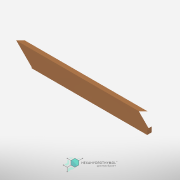
# Autodesk Inventor part: MPX-rib2
Saved by Autodesk Inventor 2016 (Build 200138000, 138)
## iProperties
Created: 2015-05-27
Part Number: MPX-rib2
Material: Wood (Cherry)
Document SubType Name: Modeling
Designer: as
Mass: 792.477 g
Surface Area: 1559.2 cm^2
Volume: 1257.9 cm^3
Density: 0.63 g/cm^3
Appearance: Cherry - Natural Low Gloss
Author: as
Autodesk Inventor part; units mm, degrees
ref_plane "YZ Plane" through (0, 0, 0) normal (1, 0, 0) x (0, 1, 0)
ref_plane "XZ Plane" through (0, 0, 0) normal (0, 1, 0) x (-1, 0, 0)
ref_plane "XY Plane" through (0, 0, 0) normal (0, 0, 1) x (1, 0, 0)
sketch "Sketch1" plane through (0, 0, 0) normal (0, 0, 1) x (1, 0, 0)
  line L0 (0, 0) -> (780, 0)
  line L1 (780, 0) -> (780, 21)
  line L2 (780, 21) -> (0, 21)
  line L3 (0, 21) -> (0, 0)
  dimension "d0" = 780
  dimension "d1" = 21
  constraints: 8 end point, 2 parallel, 1 horizontal, 1 perpendicular
  measures "d0" distance of L2.end L1.end
  measures "d1" distance of L1.end L0.end
extrude "Extrusion1" add sketch "Sketch1" along normal blind 80
sketch "Sketch2" plane through (0, 21, 0) normal (0, 1, 0) x (1, 0, 0)
  line L0 (780, 0) -> (780, -80) projected
  line L1 (780, 0) -> (680, 0)
  line L2 (680, 0) -> (680, -25)
  line L3 (680, -25) -> (780, -25)
  line L4 (780, -25) -> (780, 0)
  point P0 (0, 0)
  dimension "d4" = 100
  dimension "d5" = 25
  constraints: 8 end point, 2 parallel, 1 horizontal, 1 perpendicular
  measures "d4" distance of L3.end L2.end
  measures "d5" distance of L2.end L1.end
extrude "Extrusion2" cut sketch "Sketch2" against normal through all
body "Solid1"
